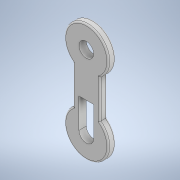
# Autodesk Inventor part: 2nd arm
Saved by Autodesk Inventor 2022 (Build 260153000, 153)
## iProperties
Created: 2022-01-28
Part Number: 2nd arm
Material: Generic
Document SubType Name: Modeling
Designer: Alexa
Density: 1 g/cm^3
Appearance: Default
Author: Alexa
Autodesk Inventor part; units mm, degrees
ref_plane "YZ Plane" through (0, 0, 0) normal (1, 0, 0) x (0, 1, 0)
ref_plane "XZ Plane" through (0, 0, 0) normal (0, 1, 0) x (-1, 0, 0)
ref_plane "XY Plane" through (0, 0, 0) normal (0, 0, 1) x (1, 0, 0)
sketch "Sketch1" plane through (0, 0, 0) normal (0, 0, 1) x (1, 0, 0)
  line L0 (0, 0) -> (20, 0)
  line L1 (20, 0) -> (20, 40.5)
  line L2 (20, 40.5) -> (0, 40.5)
  line L3 (0, 40.5) -> (0, 0)
  circle A0 centre (10, 0) radius 30
  circle A1 centre (10, 0) radius 10
  line L4 (-8, 0) -> (28, 0)
  line L5 (28, 0) -> (28, 100)
  line L6 (28, 100) -> (-8, 100)
  line L7 (-8, 100) -> (-8, 0)
  circle A2 centre (10, 100) radius 30
  circle A3 centre (10, 100) radius 10
  point P0 (28, 24)
  point P1 (28, 76)
  point P2 (-8, 76)
  point P3 (-8, 24)
  dimension "d2" = 20
  dimension "d3" = 40.5
  dimension "d4" = 60
  dimension "d5" = 20
  dimension "d6" = 36
  dimension "d7" = 100
  dimension "d8" = 60
  dimension "d9" = 20
  constraints: 16 end point, 4 centre point, 4 parallel, 2 coincident, 2 horizontal, 2 midpoint, 2 perpendicular
  measures "d2" distance of L2.end L1.end
  measures "d3" distance of L1.end L0.end
  measures "d4" diameter of A0
  measures "d5" diameter of A1
  measures "d6" distance of L6.end L5.end
  measures "d7" distance of L5.end L4.end
  measures "d8" diameter of A2
  measures "d9" diameter of A3
extrude "Extrusion1" add sketch "Sketch1" along normal blind 10 contours L4 L7 A0 L3 | L3 A0 L1 A1 | A1 L4 L5 A0 L7 | L1 A0 L5 L4 | A0 L7 A2 L5 L1 L2 L3 | L3 L2 L1 A0 | A2 L5 L6 A3 L7 | L7 L6 A3 L5 A2
fillet "Fillet1" radius 2 8 edges at (10, 130, 10) (28, 50, 10) (-8, 50, 10) (10, -30, 10) (10, 130, 0) (28, 50, 0) (10, -30, 0) (-8, 50, 0)
sketch "Sketch2" plane through (0, 0, 10) normal (0, 0, 1) x (1, 0, 0)
  line L0 (0, 0) -> (20, 0)
  line L1 (20, 0) -> (20, 40.5)
  line L2 (20, 40.5) -> (0, 40.5)
  line L3 (0, 40.5) -> (0, 0)
  dimension "d13" = 20
  dimension "d14" = 40.5
  constraints: 8 end point, 2 parallel, 1 horizontal, 1 perpendicular
  measures "d13" distance of L2.end L1.end
  measures "d14" distance of L1.end L0.end
extrude "Extrusion2" cut sketch "Sketch2" against normal blind 10.6375
body "Solid1"
